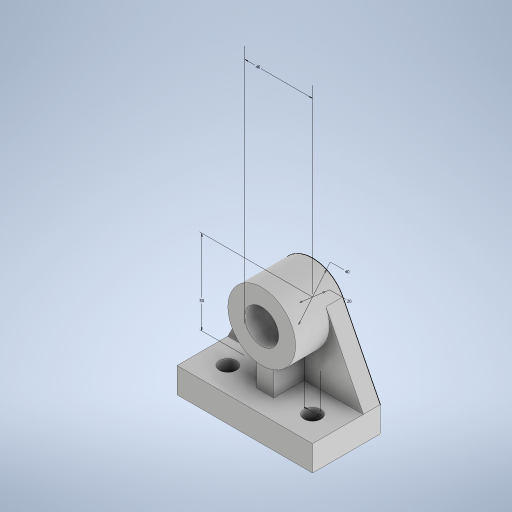
# Autodesk Inventor part: Bartosz_Zukowski_model_nr_6
Saved by Autodesk Inventor 2024 (Build 280153000, 153)
## iProperties
Created: 2024-03-20
Part Number: Bartosz_Zukowski_model_nr_6
Material: Ogólny
Document SubType Name: Modeling
Designer: student156p
Density: 1 g/cm^3
Appearance: Domyślna
Author: student156p
Autodesk Inventor part; units mm, degrees
ref_plane "YZ Plane" through (0, 0, 0) normal (1, 0, 0) x (0, 1, 0)
ref_plane "XZ Plane" through (0, 0, 0) normal (0, 1, 0) x (-1, 0, 0)
ref_plane "XY Plane" through (0, 0, 0) normal (0, 0, 1) x (1, 0, 0)
sketch "Szkic1" plane through (0, 0, 0) normal (0, 0, 1) x (1, 0, 0)
  line L0 (-40, -20) -> (40, -20)
  line L1 (40, -20) -> (40, 20)
  line L2 (40, 20) -> (-40, 20)
  line L3 (-40, 20) -> (-40, -20)
  circle A0 centre (-25, -5) radius 5
  circle A1 centre (25, -5) radius 5
  point P0 (0, 0)
  dimension "d0" = 80
  dimension "d1" = 40
  dimension "d2" = 10
  dimension "d3" = 10
  dimension "d5" = 15
  dimension "d6" = 15
  dimension "d7" = 15
  dimension "d8" = 50
  constraints: 8 end point, 2 centre point, 2 parallel, 1 horizontal, 1 perpendicular
  measures "d0" distance of L1.end L2.end
  measures "d1" distance of L0.end L1.end
  measures "d2" diameter of A0
  measures "d3" diameter of A1
  measures "d5" distance from line of L0 A1.centre
  measures "d6" distance from line of L0 A0.centre
  measures "d7" distance from line of L3 A0.centre
  measures "d8" distance of A1.centre A0.centre
extrude "Wyciągnięcie proste1" add sketch "Szkic1" along normal blind 15
sketch "Szkic3" plane through (-40, 20, 0) normal (0, 1, 0) x (1, 0, 0)
  circle A0 centre (40, 35) radius 20
  circle A1 centre (40, 35) radius 10
  line L0 (80, 0) -> (80, -15) projected
  line L1 (0, -15) -> (80, -15) projected
  line L2 (0, 0) -> (22.1342, 43.9895)
  line L3 (80, 0) -> (57.8658, 43.9895)
  line L4 (80, 0) -> (0, 0)
  line L5 (35, 0) -> (35, 15.6351)
  line L6 (45, 0) -> (45, 15.6351)
  point P0 (40, 0)
  dimension "d13" = 40
  dimension "d14" = 20
  dimension "d15" = 40
  dimension "d16" = 50
  dimension "d17" = 10
  constraints: 10 end point, 4 point on circle, 2 centre point, 2 equal length, 2 point on line, 2 tangent, 2 vertical, 1 coincident, 1 horizontal
  measures "d13" diameter of A0
  measures "d14" diameter of A1
  measures "d15" distance from line of L0 A0.centre
  measures "d16" distance from line of L1 A0.centre
  measures "d17" distance between parallel lines of L5 L6
extrude "Wyciągnięcie proste2" add sketch "Szkic3" against normal blind 30 contours A0
extrude "Wyciągnięcie proste3" add sketch "Szkic3" against normal blind 28 contours L6 L4 L5 A0
extrude "Wyciągnięcie proste4" add sketch "Szkic3" against normal blind 10 contours A0 L3 L4 L6 | A0 L5 L4 L2
